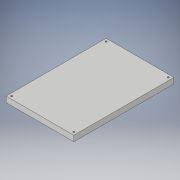
# Autodesk Inventor part: cabin_back
Saved by Autodesk Inventor 2019 (Build 230136000, 136)
## iProperties
Created: 2020-03-05
Part Number: cabin_back
Material: Generic
Document SubType Name: Modeling
Designer: laurenrhaylock
Density: 1 g/cm^3
Appearance: Default
Author: laurenrhaylock
Autodesk Inventor part; units mm, degrees
ref_plane "YZ Plane" through (0, 0, 0) normal (1, 0, 0) x (0, 1, 0)
ref_plane "XZ Plane" through (0, 0, 0) normal (0, 1, 0) x (-1, 0, 0)
ref_plane "XY Plane" through (0, 0, 0) normal (0, 0, 1) x (1, 0, 0)
sketch "Sketch1" plane through (0, 0, 0) normal (0, 1, 0) x (-1, 0, 0)
  line L0 (88.2973, 8.5512) -> (-32.2027, 8.5512)
  line L1 (-32.2027, 8.5512) -> (-32.2027, -169.4488)
  line L2 (-32.2027, -169.4488) -> (88.2973, -169.4488)
  line L3 (88.2973, -169.4488) -> (88.2973, 8.5512)
  dimension "d1" = 178
  dimension "d2" = 120.5
  constraints: 8 end point, 2 parallel, 1 horizontal, 1 perpendicular
  measures "d1" distance of L2.end L0.start
  measures "d2" distance of L0.start L0.end
extrude "Extrusion1" add sketch "Sketch1" along normal blind 10
sketch "Sketch2" plane through (0, 10, 0) normal (0, 1, 0) x (1, 0, 0)
  circle A0 centre (-83.2973, -3.5512) radius 1.5
  line L0 (-88.2973, 169.4488) -> (-88.2973, -8.5512) projected
  line L1 (-88.2973, -8.5512) -> (32.2027, -8.5512) projected
  line L2 (-88.2973, 80.4488) -> (33.9158, 80.4488)
  line L3 (32.2027, 169.4488) -> (-88.2973, 169.4488) projected
  circle A1 centre (-83.2973, 164.4488) radius 1.5
  line L4 (-28.0473, -8.5512) -> (-28.0473, 169.4488)
  line L5 (32.2027, -8.5512) -> (32.2027, 169.4488) projected
  circle A2 centre (27.2027, -3.5512) radius 1.5
  circle A3 centre (27.2027, 164.4488) radius 1.5
  point P0 (0, 0)
  dimension "d5" = 3
  dimension "d6" = 5
  dimension "d7" = 5
  dimension "d8" = 89
  dimension "d9" = 60.25
  constraints: 4 centre point, 4 end point, 3 midpoint, 3 symmetric about line, 1 horizontal, 3 other
  measures "d5" diameter of A0
  measures "d6" distance from line of L0 A0.centre
  measures "d7" distance from line of L1 A0.centre
  measures "d8" distance between parallel lines of L3 L2
  measures "d9" distance between parallel lines of L5 L4
hole "Hole1" at (-83.2973, 10, 3.5512) at (27.2027, 10, 3.5512) at (-83.2973, 10, -164.4488) at (27.2027, 10, -164.4488) direction (0, -1, 0) diameter 3 end through all
thread "Thread1" size "M3x0.5" class "6H" standard "ANSI Metric M Profile" full length
thread "Thread2" size "M3x0.5" class "6H" standard "ANSI Metric M Profile" full length
thread "Thread3" size "M3x0.5" class "6H" standard "ANSI Metric M Profile" full length
thread "Thread4" size "M3x0.5" class "6H" standard "ANSI Metric M Profile" full length
body "Solid1"
